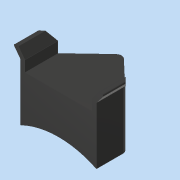
# Autodesk Inventor part: aftMount
Saved by Autodesk Inventor 2018 (Build 220112000, 112)
## iProperties
Created: 2019-09-09
Part Number: aftMount
Material: ABS Plastic
Document SubType Name: Modeling
Designer: Derek Wider
Density: 1.06 g/cm^3
Appearance: Smooth - Black
Author: Derek Wider
Autodesk Inventor part; units mm, degrees
ref_plane "YZ Plane" through (0, 0, 0) normal (1, 0, 0) x (0, 1, 0)
ref_plane "XZ Plane" through (0, 0, 0) normal (0, 1, 0) x (-1, 0, 0)
ref_plane "XY Plane" through (0, 0, 0) normal (0, 0, 1) x (1, 0, 0)
sketch "Sketch1" plane through (0, 0, 0) normal (0, 0, 1) x (1, 0, 0)
  arc A0 (22.225, 45.6803) -> (-22.225, 45.6803) centre (0, 0) ccw
  line L0 (-22.225, 45.6803) -> (-22.225, 73.66)
  line L1 (-22.225, 73.66) -> (22.225, 73.66)
  line L2 (22.225, 73.66) -> (22.225, 45.6803)
  line L3 (0, 73.66) -> (0, 50.8) construction
  line L4 (-22.225, 73.66) -> (-19.685, 73.66)
  line L5 (-19.685, 73.66) -> (-19.685, 80.01)
  line L6 (-19.685, 80.01) -> (-22.225, 80.01)
  line L7 (-22.225, 80.01) -> (-22.225, 73.66)
  line L8 (22.225, 73.66) -> (19.685, 73.66)
  line L9 (19.685, 73.66) -> (19.685, 80.01)
  line L10 (19.685, 80.01) -> (22.225, 80.01)
  line L11 (22.225, 80.01) -> (22.225, 73.66)
  dimension "d0" = 101.6
  dimension "d1" = 44.45
  dimension "d2" = 22.86
  dimension "d3" = 2.54
  dimension "d4" = 6.35
  dimension "d5" = 2.54
  dimension "d6" = 6.35
  constraints: 24 end point, 4 parallel, 4 perpendicular, 3 point on circle, 2 horizontal, 2 vertical, 1 centre point, 1 coincident, 1 horizontal alignment, 1 midpoint
  measures "d0" diameter of A0
  measures "d1" distance of L0.end L1.end
  measures "d2" distance of L3.start L3.end
  measures "d3" distance of L6.end L5.end
  measures "d4" distance of L5.end L4.end
  measures "d5" distance of L9.end L10.end
  measures "d6" distance of L8.end L9.end
extrude "Extrusion1" add sketch "Sketch1" along normal blind 38.1
sketch "Sketch2" plane through (0, 0, 38.1) normal (0, 0, 1) x (1, 0, 0)
  line L0 (-19.685, 80.01) -> (-22.225, 80.01) projected
  line L1 (-22.225, 80.01) -> (-22.225, 45.6803) projected
  line L2 (22.225, 80.01) -> (19.685, 80.01) projected
  line L3 (22.225, 45.6803) -> (22.225, 80.01) projected
  line L4 (-19.685, 80.01) -> (-23.495, 85.09)
  line L5 (-23.495, 85.09) -> (-26.67, 85.09)
  line L6 (-26.67, 85.09) -> (-22.225, 79.1633)
  line L7 (19.685, 80.01) -> (23.495, 85.09)
  line L8 (23.495, 85.09) -> (26.67, 85.09)
  line L9 (26.67, 85.09) -> (22.225, 79.1633)
  line L10 (-23.495, 85.09) -> (23.495, 85.09) construction
  line L11 (19.685, 73.66) -> (-19.685, 73.66) construction
  point P0 (0, 0)
  point P1 (0, 85.09)
  point P2 (0, 73.66)
  dimension "d9" = 2.54
  dimension "d10" = 2.54
  dimension "d11" = 5.08
  dimension "d12" = 46.99
  constraints: 14 end point, 4 point on line, 2 horizontal, 2 midpoint, 2 parallel, 1 vertical alignment
  measures "d9" distance between parallel lines of L6 L4
  measures "d10" distance between parallel lines of L7 L9
  measures "d11" distance between parallel lines of L5 L0
  measures "d12" distance of L4.end L7.end
extrude "Extrusion2" add sketch "Sketch2" against normal up to surface (38.1 mm away)
sketch "Sketch3" plane through (0, 0, 0) normal (0, 1, 0) x (-1, 0, 0)
  line L0 (0, 0) -> (26.67, 25.4)
  line L1 (26.67, 38.1) -> (26.67, 0) projected
  line L2 (26.67, 0) -> (23.495, 0) projected
  line L3 (26.67, 0) -> (26.67, 25.4)
  line L4 (26.67, 0) -> (0, 0)
  line L5 (0, 0) -> (-26.67, 25.4)
  line L6 (-26.67, 38.1) -> (-26.67, 0) projected
  line L7 (-26.67, 25.4) -> (-26.67, 0)
  line L8 (-26.67, 0) -> (0, 0)
  dimension "d15" = 25.4
  constraints: 12 end point, 2 perpendicular, 2 point on line, 2 vertical, 1 horizontal alignment
  measures "d15" distance of L1.end L0.end
extrude "Extrusion3" cut sketch "Sketch3" along normal through all
fillet "Fillet1" radius 3.175 3 edges at (0, 62.23, 0) (22.225, 62.4218, 21.1667) (-22.225, 62.4218, 21.1667)
fillet "Fillet2" radius 0.635 2 edges at (26.67, 85.09, 31.75) (-26.67, 85.09, 31.75)
equation "\"d10\" = d9"
body "Solid1"
